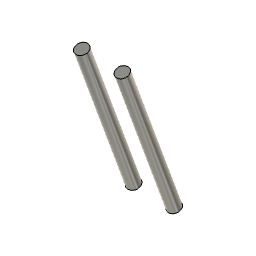
extrude_holes_example (Autodesk Fusion 360 design; units mm, degrees)
Autodesk Fusion 360 part; units mm, degrees
ref_plane "WorkPlane1" through (12.125, 0, 0) normal (0, -0.34202, 0.939693) x (1, 0, 0)
ref_plane "WorkPlane2" through (12.125, 22.2313, -61.08) normal (0, -0.34202, 0.939693) x (1, 0, 0)
sketch "Sketch1" plane through (0, 22.2313, -61.08) normal (0, -0.34202, 0.939693) x (1, 0, 0)
  circle A0 centre (20, 40) radius 6
  circle A1 centre (-20, 40) radius 6
  dimension "d3" = 12
  dimension "d4" = 40
  dimension "d5" = 40
  dimension "d6" = 20
  constraint horizontal A0.centre A1.centre
  constraint equal A0 A1
  measures "d3" diameter of A0
  measures "d4" vertical distance of origin A0.centre
  measures "d5" horizontal distance of A0.centre A1.centre
  measures "d6" horizontal distance of origin A0.centre
extrude "Extrude1" add sketch "Sketch1" along normal blind 150 makes body 1 at (25.9925, 25.336, 46.4678) makes body 2 at (-14.0075, 25.336, 46.4678)
